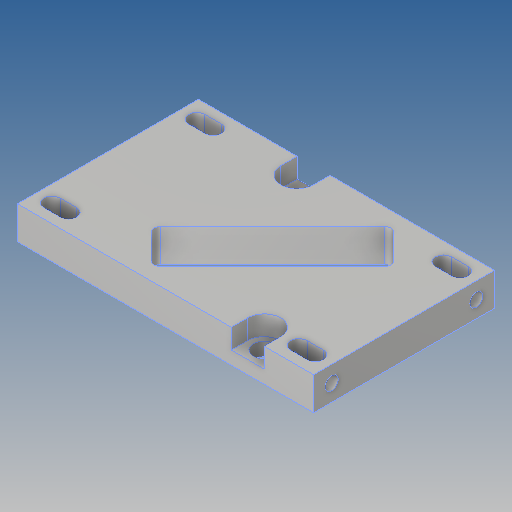
# Autodesk Inventor part: SupportGuideCarotte
Saved by Autodesk Inventor 2018 (Build 220112000, 112)
## iProperties
Created: 2022-04-27
Part Number: SupportGuideCarotte
Material: Aluminum 6061
Document SubType Name: Modeling
Designer: Nathann
Density: 2.7 g/cm^3
Appearance: Aluminum - Flat
Mass: 103.628 g
Surface Area: 135.78 cm^2
Volume: 38.3809 cm^3
Author: Nathann
Autodesk Inventor part; units mm, degrees
ref_plane "YZ Plane" through (0, 0, 0) normal (1, 0, 0) x (0, 1, 0)
ref_plane "XZ Plane" through (0, 0, 0) normal (0, 1, 0) x (-1, 0, 0)
ref_plane "XY Plane" through (0, 0, 0) normal (0, 0, 1) x (1, 0, 0)
sketch "Sketch1" plane through (0, 0, 0) normal (0, 1, 0) x (-1, 0, 0)
  line L0 (0, 0) -> (90, 0)
  line L1 (90, 0) -> (90, -55)
  line L2 (90, -55) -> (0, -55)
  line L3 (0, -55) -> (0, 0)
  dimension "d0" = 55
  dimension "d1" = 90
  constraints: 8 end point, 2 parallel, 1 horizontal, 1 perpendicular
  measures "d0" distance of L2.end L0.start
  measures "d1" distance of L1.end L2.end
extrude "Extrusion1" add sketch "Sketch1" along normal blind 10
sketch "Sketch3" plane through (0, 10, 0) normal (0, 1, 0) x (1, 0, 0)
  circle A0 centre (-20, 5) radius 3.3
  circle A1 centre (-55, 50) radius 3.3
  line L0 (-90, 0) -> (0, 0) projected
  line L1 (0, 55) -> (-90, 55) projected
  line L2 (0, 0) -> (0, 55) projected
  line L3 (-82.2074, 15) -> (-82.2074, 40) projected
  dimension "d4" = 5
  dimension "d5" = 5
  dimension "d6" = 20
  dimension "d7" = 82.2074
  dimension "d8" = 55
  dimension "d9" = 6.6
  dimension "d10" = 6.6
  constraints: 2 centre point
  measures "d4" distance from line of L0 A0.centre
  measures "d5" distance from line of L1 A1.centre
  measures "d6" distance from line of L2 A0.centre
  measures "d7" distance between parallel lines of L3 L2
  measures "d8" distance from line of L2 A1.centre
  measures "d9" diameter of A1
  measures "d10" diameter of A0
extrude "Extrusion2" cut sketch "Sketch3" against normal through all
sketch "Sketch4" plane through (0, 10, 0) normal (0, 1, 0) x (1, 0, 0)
  circle A0 centre (-20, 5) radius 3.3 projected
  circle A1 centre (-20, 5) radius 5
  line L0 (-15, 5) -> (-15, -2.6017)
  line L1 (-15, -2.6017) -> (-25, -2.6017)
  line L2 (-25, -2.6017) -> (-25, 5)
  circle A2 centre (-55, 50) radius 3.3 projected
  circle A3 centre (-55, 50) radius 5
  line L3 (0, 55) -> (-90, 55) projected
  line L4 (-50, 50) -> (-50, 57.7947)
  line L5 (-50, 57.7947) -> (-60, 57.7947)
  line L6 (-60, 57.7947) -> (-60, 50)
  point P0 (0, 0)
  dimension "d13" = 10
  constraints: 12 end point, 4 perpendicular, 4 point on circle, 2 centre point, 2 coincident, 2 vertical, 1 tangent
  measures "d13" diameter of A1
extrude "Extrusion3" cut sketch "Sketch4" against normal blind 6
sketch "Sketch5" plane through (0, 10, 0) normal (0, 1, 0) x (1, 0, 0)
  line L0 (-41.6673, 5.2261) -> (-7.7261, 39.1673) projected
  line L1 (-18.3327, 49.7739) -> (-52.2739, 15.8327) projected
  line L2 (-41.6673, 5.2261) -> (-7.7261, 39.1673) projected
  line L3 (-7.7261, 41.9957) -> (-15.5043, 49.7739) projected
  line L4 (-52.2739, 13.0043) -> (-44.4957, 5.2261) projected
  arc A0 (-52.2739, 15.8327) -> (-52.2739, 13.0043) centre (-50.8597, 14.4185) ccw projected
  line L5 (-25, 0) -> (-25, 5) projected
  arc A1 (-15, 5) -> (-25, 5) centre (-20, 5) ccw projected
  line L6 (-15, 5) -> (-15, 0) projected
  line L7 (-15, 0) -> (0, 0) projected
  line L8 (0, 0) -> (0, 55) projected
  line L9 (0, 55) -> (-50, 55) projected
  line L10 (-50, 55) -> (-50, 50) projected
  arc A2 (-60, 50) -> (-50, 50) centre (-55, 50) ccw projected
  line L11 (-60, 50) -> (-60, 55) projected
  line L12 (-60, 55) -> (-90, 55) projected
  line L13 (-90, 55) -> (-90, 0) projected
  line L14 (-90, 0) -> (-25, 0) projected
  arc A3 (-44.4957, 5.2261) -> (-41.6673, 5.2261) centre (-43.0815, 6.6403) ccw projected
  arc A4 (-15.5043, 49.7739) -> (-18.3327, 49.7739) centre (-16.9185, 48.3597) ccw projected
  arc A5 (-7.7261, 39.1673) -> (-7.7261, 41.9957) centre (-9.1403, 40.5815) ccw projected
  arc A6 (-62.2739, 15.8327) -> (-62.2739, 13.0043) centre (-60.8597, 14.4185) ccw projected
  line L15 (-28.3327, 49.7739) -> (-62.2739, 15.8327) projected
  line L16 (-62.2739, 13.0043) -> (-54.4957, 5.2261) projected
  arc A7 (-54.4957, 5.2261) -> (-51.6673, 5.2261) centre (-53.0815, 6.6403) ccw projected
  line L17 (-51.6673, 5.2261) -> (-17.7261, 39.1673) projected
  line L18 (-17.7261, 41.9957) -> (-25.5043, 49.7739) projected
  arc A8 (-25.5043, 49.7739) -> (-28.3327, 49.7739) centre (-26.9185, 48.3597) ccw projected
  arc A9 (-17.7261, 39.1673) -> (-17.7261, 41.9957) centre (-19.1403, 40.5815) ccw projected
extrude "Extrusion4" cut sketch "Sketch5" against normal through all contours L17 A7 L16 A6 L15 A8 L18 L1 A0 L4 | L4 A0 L1 L18 A9 L17
sketch "Sketch6" plane through (0, 10, 0) normal (0, 1, 0) x (1, 0, 0)
  line L0 (0, 0) -> (0, 55) projected
  line L1 (0, 27.5) -> (-90, 27.5)
  line L2 (-90, 55) -> (-90, 0) projected
  line L3 (-45, 27.5) -> (-45, 42.4026)
  line L4 (-80, 52) -> (-85, 52)
  line L5 (-85, 52) -> (-85, 47)
  line L6 (-85, 47) -> (-80, 47)
  line L7 (-80, 47) -> (-80, 52)
  circle A0 centre (-80, 49.5) radius 2.5
  circle A1 centre (-85, 49.5) radius 2.5
  line L8 (-60, 55) -> (-90, 55) projected
  line L9 (-10, 52) -> (-5, 52)
  line L10 (-5, 52) -> (-5, 47)
  line L11 (-5, 47) -> (-10, 47)
  line L12 (-10, 47) -> (-10, 52)
  circle A2 centre (-10, 49.5) radius 2.5
  circle A3 centre (-5, 49.5) radius 2.5
  line L13 (-80, 3) -> (-85, 3)
  line L14 (-85, 3) -> (-85, 8)
  line L15 (-85, 8) -> (-80, 8)
  line L16 (-80, 8) -> (-80, 3)
  circle A4 centre (-80, 5.5) radius 2.5
  circle A5 centre (-85, 5.5) radius 2.5
  line L17 (-10, 3) -> (-5, 3)
  line L18 (-5, 3) -> (-5, 8)
  line L19 (-5, 8) -> (-10, 8)
  line L20 (-10, 8) -> (-10, 3)
  circle A6 centre (-10, 5.5) radius 2.5
  circle A7 centre (-5, 5.5) radius 2.5
  dimension "d22" = 5
  dimension "d18" = 5
  dimension "d19" = 5
  dimension "d20" = 3
  dimension "d21" = 5
  constraints: 36 end point, 18 symmetric about line, 8 vertical alignment, 5 horizontal, 5 midpoint, 3 vertical, 2 parallel, 1 perpendicular, 16 other
  measures "d18" distance between parallel lines of L4 L6
  measures "d19" distance of point (-80, 49.5) point (-85, 49.5)
  measures "d20" distance between parallel lines of L8 L4
  measures "d21" distance from line of point (-85, 49.5) L2
extrude "Extrusion5" cut sketch "Sketch6" against normal through all
sketch "Sketch7" plane through (-90, 0, -55) normal (-1, 0, 0) x (0, 0, 1)
  circle A0 centre (5.5, 5) radius 2
  line L0 (0, 0) -> (0, 10) projected
  line L1 (0, 10) -> (55, 10) projected
  circle A1 centre (49.5, 5) radius 2
  line L2 (55, 0) -> (55, 10) projected
  dimension "d25" = 5.5
  dimension "d26" = 4
  dimension "d27" = 5
  dimension "d28" = 4
  dimension "d29" = 5.5
  dimension "d30" = 5
  constraints: 2 centre point
  measures "d25" distance from line of L0 A0.centre
  measures "d26" diameter of A0
  measures "d27" distance from line of L1 A0.centre
  measures "d28" diameter of A1
  measures "d29" distance from line of L2 A1.centre
  measures "d30" distance from line of L1 A1.centre
extrude "Extrusion6" cut sketch "Sketch7" against normal blind 14
sketch "Sketch8" plane through (0, 0, 0) normal (1, 0, 0) x (0, 0, -1)
  circle A0 centre (49.5, 5) radius 2 projected
  circle A1 centre (5.5, 5) radius 2 projected
  point P0 (0, 0)
extrude "Extrusion7" cut sketch "Sketch8" against normal blind 14
equation "\"d9\" = d10"
equation "\"d19\" = d22"
equation "\"d28\" = d26"
equation "\"d29\" = d25"
equation "\"d30\" = d27"
body "Solid1"
